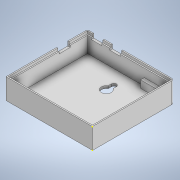
# Autodesk Inventor part: Shell 2 bottom
Saved by Autodesk Inventor 2022 (Build 260153000, 153)
## iProperties
Created: 2021-10-12
Part Number: Shell 2 bottom
Material: Generic
Document SubType Name: Modeling
Designer: Elisabeth
Density: 1 g/cm^3
Appearance: Default
Author: Elisabeth
Autodesk Inventor part; units mm, degrees
ref_plane "YZ Plane" through (0, 0, 0) normal (1, 0, 0) x (0, 1, 0)
ref_plane "XZ Plane" through (0, 0, 0) normal (0, 1, 0) x (-1, 0, 0)
ref_plane "XY Plane" through (0, 0, 0) normal (0, 0, 1) x (1, 0, 0)
sketch "Sketch1" plane through (0, 0, 0) normal (0, 1, 0) x (-1, 0, 0)
  point P0 (0, 0)
sketch "Sketch2" plane through (0, 0, 0) normal (0, 1, 0) x (-1, 0, 0)
  line L0 (0, 0) -> (70, 0)
  line L1 (70, 0) -> (70, -66)
  line L2 (70, -66) -> (0, -66)
  line L3 (0, -66) -> (0, 0)
  dimension "d0" = 70
  dimension "d1" = 66
  constraints: 8 end point, 2 parallel, 1 horizontal, 1 perpendicular
  measures "d0" distance of L1.end L2.end
  measures "d1" distance of L0.end L1.end
extrude "Extrusion1" add sketch "Sketch2" along normal blind 16.75
sketch "Sketch3" plane through (0, 16.75, 0) normal (0, 1, 0) x (1, 0, 0)
  point P0 (0, 0)
sketch "Sketch4" plane through (0, 16.75, 0) normal (0, 1, 0) x (1, 0, 0)
  line L0 (0, 66) -> (-70, 66) projected
  line L1 (-30.4814, 66) -> (-28.4814, 66)
  line L2 (-28.4814, 66) -> (-28.4814, 64)
  line L3 (-70, 66) -> (-70, 0) projected
  line L4 (-70, 37.8423) -> (-70, 39.8423)
  line L5 (-70, 39.8423) -> (-68, 39.8423)
  line L6 (-70, 0) -> (0, 0) projected
  line L7 (-28.4814, 0) -> (-30.4814, 0)
  line L8 (-30.4814, 0) -> (-30.4814, 2)
  line L9 (0, 0) -> (0, 66) projected
  line L10 (0, 38.8423) -> (0, 36.8423)
  line L11 (0, 36.8423) -> (-2, 36.8423)
  line L12 (-2, 2) -> (-60, 2)
  line L13 (-2, 64) -> (-2, 2)
  line L14 (-68, 64) -> (-68, 2)
  line L15 (-68, 64) -> (-2, 64)
  line L16 (-68, 2) -> (-2, 2)
  dimension "d5" = 2
  dimension "d6" = 2
  dimension "d7" = 2
  dimension "d8" = 2
  dimension "d9" = 2
  dimension "d10" = 2
  dimension "d11" = 2
  dimension "d12" = 2
  dimension "d102" = 2
  dimension "d103" = 2
  dimension "d104" = 2
  constraints: 26 end point, 8 point on line, 5 perpendicular, 1 parallel
  measures "d5" distance of L1.start L1.end
  measures "d6" distance of L1.end L2.end
  measures "d7" distance of L4.start L4.end
  measures "d8" distance of L4.end L5.end
  measures "d9" distance of L7.start L7.end
  measures "d10" distance of L7.end L8.end
  measures "d11" distance of L10.start L10.end
  measures "d12" distance of L10.end L11.end
  measures "d102" distance between parallel lines of L14 L3
  measures "d103" distance between parallel lines of L9 L13
  measures "d104" distance between parallel lines of L15 L0
extrude "Extrusion2" cut sketch "Sketch4" against normal blind 14.75 contours L15 L13 L12 L16 L14
sketch "Sketch10" plane through (0, 2, 0) normal (0, 1, 0) x (1, 0, 0)
  line L0 (-2, 2) -> (-68, 2) projected
  line L1 (-31, 2) -> (-48, 2)
  line L2 (-48, 2) -> (-48, 5)
  line L3 (-48, 2) -> (-63, 2)
  line L4 (-63, 2) -> (-63, 5)
  line L5 (-63, 5) -> (-48, 5)
  line L6 (-48, 5) -> (-48, 2)
  line L7 (-22, 64) -> (-7, 64)
  line L8 (-7, 64) -> (-7, 61)
  line L9 (-7, 61) -> (-22, 61)
  line L10 (-22, 61) -> (-22, 64)
  line L11 (-68, 64) -> (-2, 64) projected
  line L12 (-68, 64) -> (-68, 2)
  line L13 (-63, 2) -> (-48, 2)
  point P0 (-48, 5)
  point P1 (-63, 2)
  point P2 (-48, 2)
  dimension "d55" = 3
  dimension "d56" = 15
  dimension "d60" = 15
  dimension "d108" = 3
  constraints: 24 end point, 4 parallel, 3 horizontal, 3 perpendicular, 1 collinear, 1 vertical
  measures "d55" distance of L1.end L2.end
  measures "d56" distance of L4.end L5.end
  measures "d60" distance of L8.end L9.end
  measures "d108" distance between parallel lines of L7 L9
extrude "Extrusion5" add sketch "Sketch10" along normal blind 6
sketch "Sketch12" plane through (0, 0, 0) normal (0, -1, 0) x (1, 0, 0)
  line L0 (0, 0) -> (0, -66) projected
  arc A0 (-33, -49.6675) -> (-33, -42.7393) centre (-35, -46.2034) ccw
  arc A1 (-37, -52.3532) -> (-33, -52.3532) centre (-35, -52.3532) ccw
  line L1 (-33, -52.3532) -> (-33, -49.6675)
  line L2 (-37, -52.3532) -> (-37, -49.6675)
  arc A2 (-33, -42.7393) -> (-37, -49.6675) centre (-35, -46.2034) ccw
  constraints: 6 point on circle, 4 end point, 3 centre point, 2 tangent, 2 vertical, 1 point on line
extrude "Extrusion7" cut sketch "Sketch12" against normal blind 5
sketch "Sketch13" plane through (0, 16.75, 0) normal (0, 1, 0) x (1, 0, 0)
  line L0 (-70, 66) -> (-70, 0) projected
  line L1 (0, 0) -> (0, 66) projected
  line L2 (-69, 1) -> (-1, 1)
  line L3 (-1, 1) -> (-1, 65)
  line L4 (-1, 65) -> (-69, 65)
  line L5 (-69, 65) -> (-69, 1)
  line L6 (-70, 0) -> (0, 0) projected
  line L7 (0, 66) -> (-70, 66) projected
  line L8 (-68, 64) -> (-2, 64)
  line L9 (-2, 64) -> (-2, 2)
  line L10 (-2, 2) -> (-68, 2)
  line L11 (-68, 2) -> (-68, 64)
  dimension "d94" = 1
  dimension "d95" = 1
  dimension "d96" = 1
  dimension "d97" = 1
  dimension "d98" = 1
  dimension "d99" = 1
  dimension "d100" = 1
  dimension "d101" = 1
  constraints: 16 end point, 4 parallel, 2 horizontal, 2 perpendicular
  measures "d94" distance between parallel lines of L4 L8
  measures "d95" distance between parallel lines of L7 L4
  measures "d96" distance between parallel lines of L0 L5
  measures "d97" distance between parallel lines of L6 L2
  measures "d98" distance between parallel lines of L1 L3
  measures "d99" distance between parallel lines of L5 L11
  measures "d100" distance between parallel lines of L3 L9
  measures "d101" distance between parallel lines of L2 L10
extrude "Extrusion8" cut sketch "Sketch13" against normal blind 2 contours L5 L4 L3 L2 | L8 L9 L10 L11
sketch "Sketch15" plane through (-70, 0, -66) normal (-1, 0, 0) x (0, 0, 1)
  line L0 (62.4242, 8) -> (52.7396, 8)
  line L1 (0, 0) -> (66, 0) projected
  line L2 (0, 16.75) -> (66, 16.75) projected
  line L3 (0, 0) -> (0, 16.75) projected
  line L4 (16, 13.25) -> (25, 13.25)
  line L5 (25, 13.25) -> (25, 18.25)
  line L6 (25, 18.25) -> (16, 18.25)
  line L7 (16, 18.25) -> (16, 13.25)
  dimension "d118" = 8
  dimension "d140" = 25
  dimension "d141" = 9
  dimension "d142" = 3.5
  dimension "d143" = 5
  constraints: 10 end point, 2 horizontal, 2 parallel, 1 perpendicular
  measures "d118" distance between parallel lines of L1 L0
  measures "d140" distance between parallel lines of L3 L5
  measures "d141" distance of L4.start L4.end
  measures "d142" distance between parallel lines of L2 L4
  measures "d143" distance between parallel lines of L4 L6
extrude "Extrusion9" cut sketch "Sketch15" against normal blind 10
sketch "Sketch16" plane through (0, 0, -66) normal (0, 0, -1) x (-1, 0, 0)
  line L0 (41.4, 16.8) -> (49.9, 16.8)
  line L1 (49.9, 16.8) -> (49.9, 13.3)
  line L2 (49.9, 13.3) -> (41.4, 13.3)
  line L3 (41.4, 13.3) -> (41.4, 16.8)
  line L4 (56.5, 16.8) -> (65, 16.8)
  line L5 (65, 16.8) -> (65, 13.3)
  line L6 (65, 13.3) -> (56.5, 13.3)
  line L7 (56.5, 13.3) -> (56.5, 16.8)
  line L8 (22, 8) -> (7, 8) projected
  line L9 (70, 0) -> (70, 16.75) projected
  point P0 (0, 0)
  dimension "d127" = 8.5
  dimension "d128" = 8.5
  dimension "d129" = 3.5
  dimension "d130" = 5.3
  dimension "d131" = 28.6
  dimension "d132" = 13.5
  constraints: 16 end point, 4 parallel, 2 horizontal, 2 perpendicular, 2 point on line
  measures "d127" distance of L1.end L2.end
  measures "d128" distance of L5.end L6.end
  measures "d129" distance of L2.end L0.start
  measures "d130" distance between parallel lines of L2 L8
  measures "d131" distance between parallel lines of L3 L9
  measures "d132" distance between parallel lines of L7 L9
extrude "Extrusion10" cut sketch "Sketch16" against normal blind 10
fillet "Fillet7" radius 2 1 edges at (0, 8.375, -66)
fillet "Fillet8" radius 2 1 edges at (-70, 8.375, -66)
body "Solid1"
